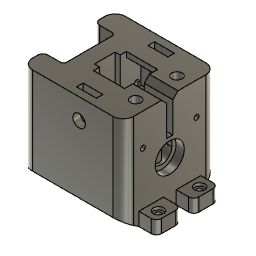
Stationary Grip Mk3 v37 (Autodesk Fusion 360 design; units mm, degrees)
Autodesk Fusion 360 part; units mm, degrees
sketch "Sketch1" plane through (0, 0, 0) normal (0, 0, 1) x (1, 0, 0)
  line L0 (0, 0) -> (70, 0)
  line L1 (70, 0) -> (70, 60)
  line L2 (70, 60) -> (0, 60)
  line L3 (0, 60) -> (0, 0)
  line L4 (70, 0) -> (95, 0)
  line L5 (95, 0) -> (95, 23.8)
  line L6 (95, 23.8) -> (70, 23.8)
  line L7 (70, 23.8) -> (70, 0)
  line L8 (70, 60) -> (95, 60)
  line L9 (95, 60) -> (95, 36.2)
  line L10 (95, 36.2) -> (70, 36.2)
  line L11 (70, 36.2) -> (70, 60)
  line L12 (0, 60) -> (-20, 60)
  line L13 (-20, 60) -> (-20, 0)
  line L14 (-20, 0) -> (0, 0)
  line L15 (0, 0) -> (0, 60)
  dimension "d1" = 60
  dimension "d77" = 70
  dimension "d116" = 25
  dimension "d117" = 23.8
  dimension "d121" = 25
  dimension "d128" = 23.8
  dimension "d229" = 20
  constraint horizontal L0
  constraint vertical L1
  constraint horizontal L2
  constraint vertical L3
  constraint coincident L0.start L3.end
  constraint horizontal L4
  constraint vertical L5
  constraint horizontal L6
  constraint vertical L7
  constraint horizontal L8
  constraint vertical L9
  constraint horizontal L10
  constraint vertical L11
  constraint horizontal L12
  constraint vertical L13
  constraint horizontal L14
  constraint vertical L15
  measures "d1" distance of L0 L2
  measures "d77" distance of L1 L3
  measures "d116" distance of L9.end L10.end
  measures "d117" distance of L8 L10
  measures "d121" distance of L5 L7
  measures "d128" distance of L4 L6
  measures "d229" distance of L3 L13
extrude "Extrude1" add sketch "Sketch1" along normal blind 10
sketch "Sketch5" plane through (0, 0, 10) normal (0, 0, 1) x (-1, 0, 0)
  line L0 (-95, -60) -> (20, -60)
  line L1 (20, 0) -> (-95, 0)
  line L2 (20, -75) -> (-78, -75)
  line L3 (-78, -75) -> (-78, 15)
  line L4 (-78, 15) -> (20, 15)
  line L5 (20, 15) -> (20, -75)
  line L6 (20, -40) -> (-78, -40)
  line L7 (-78, -40) -> (-78, -20)
  line L8 (-78, -20) -> (20, -20)
  line L9 (20, -20) -> (20, -40)
  line L10 (20, -40) -> (-15, -40)
  line L11 (-15, -40) -> (-15, -20)
  line L12 (-15, -20) -> (20, -20)
  line L13 (20, -20) -> (20, -40)
  line L14 (-70, -23.8) -> (-70, -36.2)
  line L15 (-95, 0) -> (-95, -23.8)
  line L16 (-95, -23.8) -> (-70, -23.8)
  line L17 (-70, -36.2) -> (-95, -36.2)
  line L18 (-95, -36.2) -> (-95, -60)
  line L19 (20, -60) -> (20, 0)
  line L20 (0, -75) -> (0, 15)
  line L21 (20, -60) -> (20, 0)
  line L22 (20, -55) -> (0, -55)
  line L23 (20, -5) -> (0, -5)
  dimension "d16" = 35
  dimension "d17" = 35
  dimension "d18" = 35
  dimension "d25" = 98
  dimension "d138" = 20
  dimension "d139" = 5
  dimension "d140" = 5
  constraint horizontal L2
  constraint vertical L3
  constraint horizontal L4
  constraint vertical L5
  constraint horizontal L6
  constraint vertical L7
  constraint horizontal L8
  constraint vertical L9
  constraint coincident L3 L7.end
  constraint coincident L5 L6.start
  constraint horizontal L10
  constraint vertical L11
  constraint horizontal L12
  constraint vertical L13
  constraint coincident L2 L20.start
  constraint coincident L4 L20.end
  constraint perpendicular L4 L20
  constraint coincident L21 L22.start
  constraint coincident L20 L22.end
  constraint perpendicular L20 L22
  constraint coincident L5 L23.start
  constraint coincident L20 L23.end
  constraint perpendicular L20 L23
  measures "d16" distance of L2 L6
  measures "d17" distance of L4 L8
  measures "d18" distance of L6.start L10.end
  measures "d25" distance of L3 L5
  measures "d138" distance of L20 L21
  measures "d139" distance of L0 L22
  measures "d140" distance of L1 L23
extrude "Extrude5" add sketch "Sketch5" along normal blind 85 contours L0 L3 L6 L10 L20 | L0 L2 L3 L20 | L0 L5 L19 L20 L21 L22 | L0 L2 L5 L20 | L6 L8 L10 L11 L12 L20 | L1 L3 L8 L12 L20 | L1 L3 L4 L20 | L1 L5 L19 L20 L21 L23 | L1 L4 L5 L20
sketch "Sketch6" plane through (0, 20, 0) normal (0, 1, 0) x (-1, 0, 0)
  line L0 (-78, 10) -> (-15, 10)
  line L1 (-15, 10) -> (-15, 95)
  line L2 (-15, 95) -> (-78, 95)
  line L3 (-78, 95) -> (-78, 10)
  line L4 (-20, 90) -> (-50.2, 90)
  line L5 (-50.2, 90) -> (-50.2, 59.8)
  line L6 (-50.2, 59.8) -> (-20, 59.8)
  line L7 (-20, 90) -> (-20, 59.8)
  line L8 (20, 10) -> (20, 95)
  dimension "d19" = 30.2
  dimension "d20" = 30.2
  dimension "d74" = 5
  dimension "d236" = 5
  constraint horizontal L4
  constraint vertical L5
  constraint horizontal L6
  constraint perpendicular L6 L7
  measures "d19" distance of L4.start L4.end
  measures "d20" distance of L4.start L6.end
  measures "d74" distance of L2 L4
  measures "d236" distance of L1 L7
extrude "Extrude6" cut sketch "Sketch6" along normal blind 40 and the other way blind 20 contours L4 L5 L6 L7
sketch "Sketch9" plane through (0, 0, 0) normal (0, 1, 0) x (-1, 0, 0)
  line L0 (-20, 90) -> (-50.2, 90)
  line L1 (-50.2, 90) -> (-50.2, 59.8)
  line L2 (-50.2, 59.8) -> (-20, 59.8)
  circle A0 centre (-35.1, 74.9) radius 6.1
  line L3 (-20, 59.8) -> (-20, 90)
  dimension "d36" = 12.2
  dimension "d75" = 15.1
  dimension "d100" = 15.1
  measures "d36" diameter of A0
  measures "d75" distance of L0 A0.centre
  measures "d100" distance of A0.centre L3
extrude "Extrude8" cut sketch "Sketch9" along normal blind -15 and the other way blind -75 contours A0
ref_plane "WorkPlane1" through (35.1, -1.5, 74.9) normal (0, 1, 0) x (0, 0, 1)
sketch "Sketch7" plane through (20.1, -1.5, 64.9) normal (0, 1, 0) x (1, 0, 0)
  circle A0 centre (15, -10) radius 6.1
  line L0 (5.4, -15.5426) -> (15, -21.0851)
  line L1 (15, -21.0851) -> (24.6, -15.5426)
  line L2 (24.6, -15.5426) -> (24.6, -4.4574)
  line L3 (24.6, -4.4574) -> (15, 1.0851)
  line L4 (15, 1.0851) -> (5.4, -4.4574)
  line L5 (5.4, -4.4574) -> (5.4, -15.5426)
  line L6 (24.6, -4.4574) -> (5.4, -4.4574)
  line L7 (5.4, -4.4574) -> (5.4, -30.6982)
  line L8 (5.4, -30.6982) -> (24.6, -30.6982)
  line L9 (24.6, -30.6982) -> (24.6, -4.4574)
  point P0 (15, -10)
  point P1 (15, -10)
  dimension "d136" = 9.6
  constraint coincident P0 A0.centre
  constraint horizontal L6
  constraint vertical L7
  constraint horizontal L8
  constraint vertical L9
  measures "d136" distance of P1 L5
extrude "Extrude7" cut sketch "Sketch7" against normal blind 6.3 contours A0 L0 L1 L2 L5 L6 L7 L9 | A0 L3 L4 L6 | L0 L1 L7 L8 L9
ref_plane "WorkPlane2" through (35.1, 61.5, 74.9) normal (0, -1, 0) x (0, 0, -1)
sketch "Sketch8" plane through (20.1, 61.5, 64.9) normal (0, -1, 0) x (1, 0, 0)
  circle A0 centre (15, 10) radius 6.1
  line L0 (5.4, 4.4574) -> (15, -1.0851)
  line L1 (15, -1.0851) -> (24.6, 4.4574)
  line L2 (24.6, 4.4574) -> (24.6, 15.5426)
  line L3 (24.6, 15.5426) -> (15, 21.0851)
  line L4 (15, 21.0851) -> (5.4, 15.5426)
  line L5 (5.4, 15.5426) -> (5.4, 4.4574)
  line L6 (24.6, 4.4574) -> (5.4, 4.4574)
  line L7 (5.4, 4.4574) -> (5.4, 31.3232)
  line L8 (5.4, 31.3232) -> (24.6, 31.3232)
  line L9 (24.6, 31.3232) -> (24.6, 4.4574)
  point P0 (15, 10)
  point P1 (15, 10)
  dimension "d137" = 9.6
  constraint coincident P0 A0.centre
  constraint horizontal L6
  constraint vertical L7
  constraint horizontal L8
  constraint vertical L9
  measures "d137" distance of P1 L5
extrude "Extrude9" cut sketch "Sketch8" against normal blind 6.3 contours A0 L2 L3 L4 L5 L6 L7 L9 | A0 L0 L1 L6 | L3 L4 L7 L8 L9
sketch "Sketch10" plane through (0, 0, 10) normal (0, 0, 1) x (-1, 0, 0)
  line L0 (-78, -40) -> (-15, -40)
  line L1 (-15, -40) -> (-15, -20)
  line L2 (-15, -20) -> (-78, -20)
  circle A0 centre (-25, -30) radius 2.6
  circle A1 centre (-87, -50) radius 2.6
  circle A2 centre (-55, -30) radius 2.6
  circle A3 centre (-87, -10) radius 2.6
  circle A4 centre (-40, -30) radius 2.6
  line L3 (-70, -23.8) -> (-70, -36.2)
  line L4 (-95, -36.2) -> (-95, -60)
  line L5 (-95, 0) -> (-95, -23.8)
  line L6 (-15, -20) -> (-15, -40)
  line L7 (-78, -20) -> (-78, 0)
  line L8 (-78, 0) -> (-95, 0)
  line L9 (-95, 0) -> (-95, -23.8)
  line L10 (-95, -23.8) -> (-70, -23.8)
  line L11 (-70, -36.2) -> (-95, -36.2)
  line L12 (-95, -36.2) -> (-95, -60)
  line L13 (-95, -60) -> (-78, -60)
  line L14 (-78, -60) -> (-78, -40)
  line L15 (20, -5) -> (0, -5)
  line L16 (0, -5) -> (0, -55)
  line L17 (0, -55) -> (20, -55)
  line L18 (20, -55) -> (20, -5)
  circle A5 centre (10, -50) radius 2.6
  circle A6 centre (10, -30) radius 2.6
  circle A7 centre (10, -10) radius 2.6
  line L19 (0, -5) -> (20, -5)
  line L20 (20, -55) -> (0, -55)
  dimension "d45" = 5.2
  dimension "d46" = 5.2
  dimension "d49" = 5.2
  dimension "d51" = 5.2
  dimension "d102" = 5.2
  dimension "d120" = 15
  dimension "d122" = 10
  dimension "d123" = 15
  dimension "d131" = 8
  dimension "d141" = 5.2
  dimension "d142" = 5.2
  dimension "d143" = 5.2
  dimension "d144" = 5
  dimension "d145" = 25
  dimension "d146" = 5
  measures "d45" diameter of A0
  measures "d46" diameter of A1
  measures "d49" diameter of A2
  measures "d51" diameter of A3
  measures "d102" diameter of A4
  measures "d120" distance of A2.centre L3
  measures "d122" distance of A0.centre L6
  measures "d123" distance of A0.centre A4.centre
  measures "d131" distance of A3.centre L5
  measures "d141" diameter of A5
  measures "d142" diameter of A6
  measures "d143" diameter of A7
  measures "d144" distance of A7.centre L19
  measures "d145" distance of A6.centre L20
  measures "d146" distance of A5.centre L20
extrude "Extrude10" cut sketch "Sketch10" against normal blind 10 contours A0 | A1 | A2 | A3 | A4 | A5 | A6 | A7
sketch "Sketch11" plane through (50.2, 0, 0) normal (-1, 0, 0) x (0, -1, 0)
  line L0 (-40, 59.8) -> (-40, 90)
  line L1 (-40, 90) -> (-60, 90)
  line L2 (-60, 90) -> (-60, 59.8)
  line L3 (-60, 59.8) -> (-40, 59.8)
  line L4 (-20, 90) -> (-20, 59.8)
  line L5 (-20, 59.8) -> (0, 59.8)
  line L6 (0, 59.8) -> (0, 90)
  line L7 (0, 90) -> (-20, 90)
  line L8 (-40, 59.8) -> (-33, 59.8)
  line L9 (-33, 59.8) -> (-33, 95)
  line L10 (-33, 95) -> (-40, 95)
  line L11 (-40, 95) -> (-40, 59.8)
  line L12 (-20, 59.8) -> (-27, 59.8)
  line L13 (-27, 59.8) -> (-27, 95)
  line L14 (-27, 95) -> (-20, 95)
  line L15 (-20, 95) -> (-20, 59.8)
  line L16 (15, 95) -> (-20, 95)
  line L17 (-40, 95) -> (-75, 95)
  line L18 (-40, 59.8) -> (-20, 59.8)
  line L19 (-20, 59.8) -> (-20, 54.8)
  line L20 (-20, 54.8) -> (-40, 54.8)
  line L21 (-40, 54.8) -> (-40, 59.8)
  line L22 (-40, 10) -> (-40, 95)
  line L23 (-20, 10) -> (-20, 95)
  line L24 (-27, 54.8) -> (-20, 47.8)
  line L25 (-33, 54.8) -> (-40, 47.8)
  dimension "d54" = 7
  dimension "d55" = 7
  dimension "d176" = 5
  dimension "d177" = 135
  dimension "d178" = 45
  dimension "d179" = 7
  dimension "d180" = 7
  constraint horizontal L8
  constraint vertical L9
  constraint horizontal L10
  constraint vertical L11
  constraint coincident L0.start L3.end
  constraint horizontal L12
  constraint vertical L13
  constraint horizontal L14
  constraint vertical L15
  constraint coincident L4.end L5.start
  constraint collinear L14 L16
  constraint horizontal L18
  constraint vertical L19
  constraint horizontal L20
  constraint vertical L21
  constraint coincident L20 L24.start
  constraint coincident L23 L24.end
  constraint coincident L20 L25.start
  constraint coincident L22 L25.end
  measures "d54" distance of L13 L15
  measures "d55" distance of L9 L11
  measures "d176" distance of L0.start L20.end
  measures "d177" angle of L20 L25
  measures "d178" angle of L20 L24
  measures "d179" distance of L22 L25.start
  measures "d180" distance of L23 L24.start
extrude "Extrude11" add sketch "Sketch11" against normal blind 27.8 contours L0 L8 L9 L10 L11 L18 L22 | L8 L12 L18 L19 L20 L21 L22 L23 | L20 L22 L25 | L4 L12 L13 L14 L15 L18 L23 | L20 L23 L24
sketch "Sketch23" plane through (0, 0, 59.8) normal (0, 0, 1) x (-1, 0, 0)
  line L0 (-50.2, -33) -> (-50.2, -27)
  line L1 (-50.2, -27) -> (-78, -27)
  line L2 (-78, -27) -> (-78, -33)
  line L3 (-78, -33) -> (-50.2, -33)
  line L4 (-50.2, -33) -> (-60.2, -33)
  line L5 (-60.2, -33) -> (-60.2, -27)
  line L6 (-60.2, -27) -> (-50.2, -27)
  line L7 (-50.2, -27) -> (-50.2, -33)
  dimension "d182" = 10
  constraint horizontal L4
  constraint vertical L5
  constraint horizontal L6
  constraint vertical L7
  constraint coincident L0.start L3.end
  measures "d182" distance of L0.start L4.end
extrude "Extrude25" cut sketch "Sketch23" against normal blind 6 contours L0 L1 L3 L4 L5 L6 L7
chamfer "Chamfer19" distance 4 angle 45 1 edges at (60.2, 30, 59.8)
chamfer "Chamfer10" distance 15 distance2 10 2 edges at (29, 0, 10) (29, 60, 10) measured on face at (45.3333, -5, 10) measured on face at (45.3333, 65, 10)
sketch "Sketch21" plane through (78, 0, 0) normal (1, 0, 0) x (0, 1, 0)
  line L0 (0, 10) -> (20, 10)
  line L1 (20, 10) -> (20, 47.8)
  line L2 (75, 95) -> (33, 95)
  line L3 (-15, 95) -> (-15, 10)
  line L4 (-15, 10) -> (0, 0)
  line L5 (0, 0) -> (0, 10)
  circle A0 centre (30, 43) radius 14.1
  line L6 (0, 0) -> (23.8, 0)
  line L7 (27, 59.8) -> (27, 95)
  line L8 (20, 47.8) -> (27, 54.8)
  line L9 (27, 54.8) -> (33, 54.8)
  line L10 (33, 54.8) -> (40, 47.8)
  line L11 (40, 47.8) -> (40, 10)
  line L12 (40, 10) -> (60, 10)
  line L13 (60, 10) -> (60, 0)
  line L14 (60, 0) -> (75, 10)
  line L15 (75, 10) -> (75, 95)
  line L16 (33, 95) -> (33, 59.8)
  line L17 (33, 59.8) -> (27, 59.8)
  line L18 (27, 95) -> (-15, 95)
  dimension "d157" = 28.2
  dimension "d158" = 43
  measures "d157" diameter of A0
  measures "d158" distance of A0.centre L6
extrude "Extrude21" cut sketch "Sketch21" against normal blind 8 contours L1 A0 L8 L9 L10 L11 | L1 A0 L8 L9 L10 L11
sketch "Sketch18" plane through (70, 0, 0) normal (1, 0, 0) x (0, 1, 0)
  line L0 (-15, 95) -> (-15, 10)
  line L1 (0, 10) -> (20, 10)
  line L2 (20, 10) -> (20, 33.0597)
  line L3 (27, 95) -> (-15, 95)
  line L4 (47.5, 10) -> (12.5, 10)
  line L5 (12.5, 10) -> (12.5, 43)
  line L6 (47.5, 43) -> (47.5, 10)
  line L7 (-15, 10) -> (0, 0)
  line L8 (0, 0) -> (0, 10)
  line L9 (75, 10) -> (75, 95)
  line L10 (40, 33.0597) -> (40, 10)
  line L11 (60, 10) -> (60, 0)
  line L12 (60, 0) -> (75, 10)
  arc A0 (40, 33.0597) -> (20, 33.0597) centre (30, 43) ccw
  circle A1 centre (30, 43) radius 17.5
  circle A2 centre (30, 43) radius 14.1
  line L13 (27, 59.8) -> (27, 95)
  line L14 (40, 10) -> (60, 10)
  line L15 (75, 95) -> (33, 95)
  line L16 (33, 95) -> (33, 59.8)
  line L17 (33, 59.8) -> (27, 59.8)
  dimension "d230" = 35
  constraint horizontal L4
  constraint vertical L5
  constraint vertical L6
  constraint concentric A0 A1
  constraint coincident L6.start A1
  constraint tangent L5 A1
  constraint tangent L6 A1
  constraint coincident L5.end A1
  constraint concentric A0 A2
  measures "d230" diameter of A1
extrude "Extrude22" add sketch "Sketch18" 1 faces at (70, 27.9333, 3.3333) along normal blind 8 contours L2 L10 A0 A1 A2 L13 L16 L17 | A1 L13 L16 L17 | L1 L2 L4 L5 A1 | L2 L4 L10 A1 | L2 L10 A1 A2
sketch "Sketch22" plane through (0, 0, 10) normal (0, 0, 1) x (-1, 0, 0)
  line L0 (-70, -20) -> (-70, -40)
  line L1 (-70, -40) -> (-15, -40)
  line L2 (-15, -40) -> (-15, -20)
  line L3 (-15, -20) -> (-70, -20)
  circle A0 centre (-55, -30) radius 2.6
  circle A1 centre (-40, -30) radius 2.6
  circle A2 centre (-25, -30) radius 2.6
  circle A3 centre (10, -50) radius 2.6
  circle A4 centre (10, -30) radius 2.6
  circle A5 centre (10, -10) radius 2.6
  line L4 (20, -5) -> (0, -5)
  line L5 (0, -5) -> (0, -55)
  line L6 (0, -55) -> (20, -55)
  line L7 (20, -55) -> (20, -5)
  circle A6 centre (-25, -30) radius 5
  circle A7 centre (-40, -30) radius 5
  circle A8 centre (-55, -30) radius 5
  circle A9 centre (10, -50) radius 5
  circle A10 centre (10, -30) radius 5
  circle A11 centre (10, -10) radius 5
  circle A12 centre (-87, -50) radius 2.6
  line L8 (-78, -60) -> (-78, -36.2)
  line L9 (-78, -36.2) -> (-95, -36.2)
  line L10 (-95, -36.2) -> (-95, -60)
  line L11 (-95, -60) -> (-78, -60)
  circle A13 centre (-87, -10) radius 2.6
  line L12 (-78, -23.8) -> (-78, 0)
  line L13 (-78, 0) -> (-95, 0)
  line L14 (-95, 0) -> (-95, -23.8)
  line L15 (-95, -23.8) -> (-78, -23.8)
  circle A14 centre (-87, -50) radius 5
  circle A15 centre (-87, -10) radius 5
  dimension "d163" = 10
  dimension "d164" = 10
  dimension "d165" = 10
  dimension "d166" = 10
  dimension "d167" = 10
  dimension "d168" = 10
  dimension "d169" = 10
  dimension "d170" = 10
  constraint concentric A2 A6
  constraint concentric A1 A7
  constraint concentric A0 A8
  constraint concentric A3 A9
  constraint concentric A4 A10
  constraint concentric A5 A11
  constraint concentric A12 A14
  constraint concentric A13 A15
  measures "d163" diameter of A6
  measures "d164" diameter of A7
  measures "d165" diameter of A8
  measures "d166" diameter of A9
  measures "d167" diameter of A10
  measures "d168" diameter of A11
  measures "d169" diameter of A14
  measures "d170" diameter of A15
extrude "Extrude23" add sketch "Sketch22" along normal blind 5 contours L0 L1 L2 L3 | L4 L5 L6 L7
extrude "Extrude24" add sketch "Sketch22" along normal blind 2.8 contours L8 L9 L10 L11 | L12 L13 L14 L15
sketch "Sketch12" plane through (0, 0, 95) normal (0, 0, 1) x (-1, 0, 0)
  line L0 (-15, -20) -> (-15, -40)
  line L1 (-15, -40) -> (-50.2, -40)
  line L2 (-50.2, -40) -> (-50.2, -33)
  line L3 (-50.2, -33) -> (-78, -33)
  line L4 (-78, -75) -> (20, -75)
  line L5 (20, -75) -> (20, -55)
  line L6 (20, 15) -> (-78, 15)
  line L7 (-78, -27) -> (-50.2, -27)
  line L8 (-20, -46) -> (-50.2, -46)
  line L9 (-50.2, -46) -> (-50.2, -14)
  line L10 (-50.2, -14) -> (-20, -14)
  line L11 (-20, -14) -> (-20, -46)
  line L12 (-44.7, -61.5) -> (-25.5, -61.5)
  line L13 (-25.5, -67.8) -> (-44.7, -67.8)
  line L14 (-25.5, 1.5) -> (-44.7, 1.5)
  line L15 (-44.7, 7.8) -> (-25.5, 7.8)
  line L16 (-50.2, -20) -> (-15, -20)
  line L17 (-78, -33) -> (-78, -75)
  line L18 (-44.7, 1.5) -> (-44.7, 7.8)
  line L19 (-25.5, 7.8) -> (-25.5, 1.5)
  line L20 (-25.5, -61.5) -> (-25.5, -67.8)
  line L21 (-44.7, -67.8) -> (-44.7, -61.5)
  line L22 (0, -55) -> (0, -5)
  line L23 (20, -55) -> (0, -55)
  line L24 (0, -5) -> (20, -5)
  line L25 (-78, 15) -> (-78, -27)
  line L26 (-50.2, -27) -> (-50.2, -20)
  line L27 (20, -5) -> (20, 15)
  dimension "d64" = 32
  dimension "d67" = 6
  dimension "d101" = 5
  constraint horizontal L8
  constraint vertical L9
  constraint horizontal L10
  constraint vertical L11
  constraint collinear L2 L9
  measures "d64" distance of L8.start L10.end
  measures "d67" distance of L1 L8
  measures "d101" distance of L0 L11
extrude "Extrude12" cut sketch "Sketch12" against normal blind 5 contours L9 L10 L11 L16 | L1 L2 L9 L11 L16 L26 | L1 L8 L9 L11
sketch "Sketch13" plane through (0, 0, 0) normal (-1, 0, 0) x (0, -1, 0)
  line L0 (15, 95) -> (-5, 95)
  circle A0 centre (-30, 43) radius 7
  line L1 (15, 10) -> (15, 95)
  line L2 (-75, 95) -> (-75, 10)
  line L3 (-60, 0) -> (0, 0)
  line L4 (0, 0) -> (15, 10)
  line L5 (-5, 95) -> (-5, 10)
  line L6 (-5, 10) -> (-55, 10)
  line L7 (-55, 10) -> (-55, 95)
  line L8 (-55, 95) -> (-75, 95)
  line L9 (-75, 10) -> (-60, 0)
  line L10 (-5, 15) -> (-5, 95)
  line L11 (-5, 95) -> (-55, 95)
  line L12 (-55, 95) -> (-55, 15)
  line L13 (-55, 15) -> (-5, 15)
  line L14 (-60, 0) -> (0, 0)
  dimension "d69" = 14
  dimension "d231" = 43
  measures "d69" diameter of A0
  measures "d231" distance of A0.centre L14
extrude "Extrude13" cut sketch "Sketch13" against normal blind 15 contours A0
sketch "Sketch19" plane through (70, 0, 0) normal (-1, 0, 0) x (0, -1, 0)
  line L0 (-20, 10) -> (-20, 33.0597)
  arc A0 (-40, 33.0597) -> (-20, 33.0597) centre (-30, 43) ccw
  line L1 (-40, 33.0597) -> (-40, 10)
  line L2 (-40, 10) -> (-20, 10)
  circle A1 centre (-30, 43) radius 10
  line L3 (-40, 10) -> (-40, 43)
  line L4 (-20, 10) -> (-20, 43)
  line L5 (-20, 15) -> (-20, 33.0597)
  arc A2 (-40, 33.0597) -> (-20, 33.0597) centre (-30, 43) ccw
  line L6 (-40, 33.0597) -> (-40, 15)
  line L7 (-40, 15) -> (-20, 15)
  dimension "d132" = 20
  constraint concentric A0 A1
  constraint coincident L1.end L2.start
  constraint coincident A1 L3.end
  constraint tangent A1 L3
  constraint coincident L0.start L2.end
  constraint coincident A1 L4.end
  constraint tangent A1 L4
  measures "d132" diameter of A1
extrude "Extrude18" add sketch "Sketch19" along normal blind 3 contours L0 L1 L2 L3 L4 L7 | L0 A0 L1 L3 L4 L5 A2 L6 L7 | A0 A1 L3 L4 A2
chamfer "Chamfer11" distance 5 angle 45 2 edges at (64.1, 33, 95) (64.1, 27, 95)
fillet "Fillet4" radius 10 4 edges at (78, -15, 52.5) (-20, -15, 52.5) (-20, 75, 52.5) (78, 75, 52.5)
fillet "Fillet5" radius 5 4 edges at (95, 60, 5) (95, 36.2, 5) (95, 23.8, 5) (95, 0, 5)
fillet "Fillet6" radius 5 2 edges at (-20, 55, 52.5) (-20, 5, 52.5)
chamfer "Chamfer14" distance 2 angle 45 3 edges at (0, 5, 55) (0, 55, 55) (0, 30, 15)
chamfer "Chamfer15" distance 7 angle 45 4 edges at (67, 40, 29) (67, 20, 29) (50.2, 20, 53.8) (50.2, 40, 53.8)
fillet "Fillet8" radius 5 1 edges at (70, 30, 59.8)
sketch "Sketch24" plane through (0, 0, 95) normal (0, 0, 1) x (-1, 0, 0)
  line L0 (-25.5, -61.5) -> (-25.5, -67.8)
  line L1 (-25.5, -67.8) -> (-44.7, -67.8)
  line L2 (-44.7, -67.8) -> (-44.7, -61.5)
  line L3 (-44.7, -61.5) -> (-25.5, -61.5)
  line L4 (-44.7, 1.5) -> (-44.7, 7.8)
  line L5 (-44.7, 7.8) -> (-25.5, 7.8)
  line L6 (-25.5, 7.8) -> (-25.5, 1.5)
  line L7 (-25.5, 1.5) -> (-44.7, 1.5)
  arc A0 (15, -5) -> (20, 0) centre (15, 0) ccw
  line L8 (20, 0) -> (20, 5)
  arc A1 (20, 5) -> (10, 15) centre (10, 5) ccw
  line L9 (10, 15) -> (-68, 15)
  arc A2 (-68, 15) -> (-78, 5) centre (-68, 5) ccw
  line L10 (-78, 5) -> (-78, -22)
  line L11 (-78, -22) -> (-50.2, -22)
  line L12 (-50.2, -22) -> (-50.2, -14)
  line L13 (-50.2, -14) -> (-20, -14)
  line L14 (-20, -14) -> (-20, -20)
  line L15 (-20, -20) -> (-15, -20)
  line L16 (-15, -20) -> (-15, -40)
  line L17 (-15, -40) -> (-20, -40)
  line L18 (-20, -40) -> (-20, -46)
  line L19 (-20, -46) -> (-50.2, -46)
  line L20 (-50.2, -46) -> (-50.2, -38)
  line L21 (-50.2, -38) -> (-78, -38)
  line L22 (-78, -38) -> (-78, -65)
  arc A3 (-78, -65) -> (-68, -75) centre (-68, -65) ccw
  line L23 (-68, -75) -> (10, -75)
  arc A4 (10, -75) -> (20, -65) centre (10, -65) ccw
  line L24 (20, -65) -> (20, -60)
  arc A5 (20, -60) -> (15, -55) centre (15, -60) ccw
  line L25 (15, -55) -> (2, -55)
  line L26 (2, -55) -> (0, -53)
  line L27 (0, -53) -> (0, -7)
  line L28 (0, -7) -> (2, -5)
  line L29 (2, -5) -> (15, -5)
  circle A6 centre (-65, -10) radius 2.6
  circle A7 centre (-65, -50) radius 2.6
  dimension "d186" = 5.2
  dimension "d187" = 5.2
  dimension "d232" = 25
  dimension "d233" = 25
  dimension "d234" = 13
  dimension "d235" = 13
  measures "d186" diameter of A6
  measures "d187" diameter of A7
  measures "d232" distance of L9 A6.centre
  measures "d233" distance of L23 A7.centre
  measures "d234" distance of L10 A6.centre
  measures "d235" distance of L22 A7.centre
extrude "Extrude26" cut sketch "Sketch24" against normal blind 95 contours A6 | A7
sketch "Sketch25" plane through (0, 0, 95) normal (0, 0, 1) x (-1, 0, 0)
  circle A0 centre (-65, -50) radius 2.6
  circle A1 centre (-65, -10) radius 2.6
  line L0 (-25.5, -61.5) -> (-25.5, -67.8)
  line L1 (-25.5, -67.8) -> (-44.7, -67.8)
  line L2 (-44.7, -67.8) -> (-44.7, -61.5)
  line L3 (-44.7, -61.5) -> (-25.5, -61.5)
  line L4 (-44.7, 1.5) -> (-44.7, 7.8)
  line L5 (-44.7, 7.8) -> (-25.5, 7.8)
  line L6 (-25.5, 7.8) -> (-25.5, 1.5)
  line L7 (-25.5, 1.5) -> (-44.7, 1.5)
  arc A2 (15, -5) -> (20, 0) centre (15, 0) ccw
  line L8 (20, 0) -> (20, 5)
  arc A3 (20, 5) -> (10, 15) centre (10, 5) ccw
  line L9 (10, 15) -> (-68, 15)
  arc A4 (-68, 15) -> (-78, 5) centre (-68, 5) ccw
  line L10 (-78, 5) -> (-78, -22)
  line L11 (-78, -22) -> (-50.2, -22)
  line L12 (-50.2, -22) -> (-50.2, -14)
  line L13 (-50.2, -14) -> (-20, -14)
  line L14 (-20, -14) -> (-20, -20)
  line L15 (-20, -20) -> (-15, -20)
  line L16 (-15, -20) -> (-15, -40)
  line L17 (-15, -40) -> (-20, -40)
  line L18 (-20, -40) -> (-20, -46)
  line L19 (-20, -46) -> (-50.2, -46)
  line L20 (-50.2, -46) -> (-50.2, -38)
  line L21 (-50.2, -38) -> (-78, -38)
  line L22 (-78, -38) -> (-78, -65)
  arc A5 (-78, -65) -> (-68, -75) centre (-68, -65) ccw
  line L23 (-68, -75) -> (10, -75)
  arc A6 (10, -75) -> (20, -65) centre (10, -65) ccw
  line L24 (20, -65) -> (20, -60)
  arc A7 (20, -60) -> (15, -55) centre (15, -60) ccw
  line L25 (15, -55) -> (2, -55)
  line L26 (2, -55) -> (0, -53)
  line L27 (0, -53) -> (0, -7)
  line L28 (0, -7) -> (2, -5)
  line L29 (2, -5) -> (15, -5)
  circle A8 centre (-65, -50) radius 5
  circle A9 centre (-65, -10) radius 5
  dimension "d190" = 10
  dimension "d191" = 10
  constraint concentric A0 A8
  constraint concentric A1 A9
  measures "d190" diameter of A8
  measures "d191" diameter of A9
extrude "Extrude27" cut sketch "Sketch25" against normal blind 10 contours A8 | A9
sketch "Sketch27" plane through (-20, 0, 0) normal (-1, 0, 0) x (0, -1, 0)
  line L0 (0, 95) -> (0, 15)
  line L1 (0, 15) -> (-60, 15)
  line L2 (-60, 15) -> (-60, 95)
  line L3 (-60, 95) -> (-65, 95)
  line L4 (-65, 95) -> (-65, 3.3333)
  line L5 (-65, 3.3333) -> (-60, 0)
  line L6 (-60, 0) -> (0, 0)
  line L7 (0, 0) -> (5, 3.3333)
  line L8 (5, 3.3333) -> (5, 95)
  line L9 (5, 95) -> (0, 95)
  circle A0 centre (-56, 63.8) radius 2.4
  circle A1 centre (-4, 63.8) radius 2.4
  line L10 (15, 10) -> (15, 95)
  line L11 (-75, 95) -> (-75, 10)
  line L12 (-33, 59.8) -> (-60, 59.8)
  line L13 (-60, 59.8) -> (-40, 59.8)
  line L14 (-40, 59.8) -> (-33, 59.8)
  line L15 (-20, 59.8) -> (0, 59.8)
  line L16 (0, 59.8) -> (-27, 59.8)
  line L17 (-27, 59.8) -> (-20, 59.8)
  circle A2 centre (-56, 63.8) radius 5
  circle A3 centre (-4, 63.8) radius 5
  dimension "d204" = 4.8
  dimension "d205" = 4.8
  dimension "d206" = 19
  dimension "d207" = 19
  dimension "d209" = 4
  dimension "d210" = 4
  dimension "d213" = 10
  dimension "d214" = 10
  constraint concentric A0 A2
  constraint concentric A1 A3
  measures "d204" diameter of A0
  measures "d205" diameter of A1
  measures "d206" distance of A1.centre L10
  measures "d207" distance of A0.centre L11
  measures "d209" distance of A1.centre L15
  measures "d210" distance of A0.centre L12
  measures "d213" diameter of A2
  measures "d214" diameter of A3
extrude "Extrude29" cut sketch "Sketch27" against normal blind 98 contours A0 | A1
extrude "Extrude30" cut sketch "Sketch27" against normal blind 8 contours L0 L15 L16 A3 | L0 A3 | L15 L16 A3 | L2 A2 | L2 L12 L13 A2 | L12 L13 A2 picked at (-3.9402, 60.3356) picked at (-56.0598, 60.3356)
extrude "Extrude31" add sketch "Sketch27" along normal blind -20 and the other way blind 8 contours L0 L15 L16 A3 | L0 A3 | L15 L16 A3 | L2 A2 | L2 L12 L13 A2 | L12 L13 A2 picked at (-3.9402, 60.3356) picked at (-56.0598, 60.3356)
fillet "Fillet9" radius 4 4 edges at (-7, 55, 58.901) (-7, 55, 68.699) (-7, 5, 68.699) (-7, 5, 58.901)
chamfer "Chamfer20" distance 1 angle 45 2 edges at (0, 51, 63.8) (0, 9, 63.8)
chamfer "Chamfer21" distance 0.4 angle 45 2 edges at (-12, 58.2376, 62.9321) (-12, 6.2376, 62.9321)
